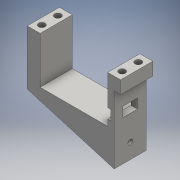
# Autodesk Inventor part: supportservopetitrobot
Saved by Autodesk Inventor 2016 (Build 200138000, 138)
## iProperties
Created: 2017-04-12
Part Number: supportservopetitrobot
Material: Générique
Document SubType Name: Modeling
Designer: Galileo
Density: 1 g/cm^3
Appearance: Par défaut
Author: Galileo
Autodesk Inventor part; units mm, degrees
ref_plane "YZ Plane" through (0, 0, 0) normal (1, 0, 0) x (0, 1, 0)
ref_plane "XZ Plane" through (0, 0, 0) normal (0, 1, 0) x (-1, 0, 0)
ref_plane "XY Plane" through (0, 0, 0) normal (0, 0, 1) x (1, 0, 0)
sketch "Esquisse1" plane through (0, 0, 0) normal (0, 1, 0) x (-1, 0, 0)
  line L0 (0, 0) -> (0, -8)
  line L1 (0, 0) -> (8, 0)
  line L2 (8, 0) -> (8, -29)
  line L3 (8, -29) -> (50, -29)
  line L4 (50, -29) -> (50, 0)
  line L5 (0, -8) -> (4, -8)
  line L6 (4, -8) -> (4, -50)
  line L7 (50, 0) -> (58, 0)
  line L8 (58, 0) -> (58, -34)
  line L9 (58, -34) -> (4, -50)
  dimension "d0" = 8
  dimension "d1" = 29
  dimension "d2" = 42
  dimension "d3" = 8
  dimension "d4" = 42
  dimension "d5" = 8
  dimension "d6" = 34
  dimension "d11" = 4
  dimension "d12" = 29
  constraints: 20 end point, 4 horizontal, 3 vertical, 2 perpendicular
  measures "d0" distance of L0.start L1.end
  measures "d1" distance of L1.end L2.end
  measures "d2" distance of L2.end L3.end
  measures "d3" distance of L0.start L0.end
  measures "d4" distance of L5.end L6.end
  measures "d5" distance of L4.end L7.end
  measures "d6" distance of L7.end L8.end
  measures "d11" distance of L0.end L5.end
  measures "d12" distance of L3.end L4.end
extrude "Extrusion1" add sketch "Esquisse1" along normal blind 20
sketch "Esquisse2" plane through (-58, 0, 0) normal (0, 0, 1) x (1, 0, 0)
  line L0 (0, 20) -> (8, 20) projected
  line L1 (0, 0) -> (8, 0) projected
  line L2 (0, 0) -> (0, 20) projected
  point P0 (58, 0)
  point P1 (4, 15)
  point P2 (4, 5)
  dimension "d15" = 10
  dimension "d17" = 5
  dimension "d18" = 4
  dimension "d19" = 4
  measures "d15" distance of point (4, 5) point (4, 15)
  measures "d17" distance from line of L1 point (4, 5)
  measures "d18" distance from line of L2 point (4, 15)
  measures "d19" distance from line of L2 point (4, 5)
hole "Perçage1" at (-54, 15, 0) at (-54, 5, 0) direction (0, 0, -1) diameter 4 depth 10 tip angle 118
sketch "Esquisse3" plane through (-8, 0, 0) normal (0, 0, 1) x (1, 0, 0)
  line L0 (0, 20) -> (8, 20) projected
  line L1 (8, 0) -> (8, 20) projected
  point P0 (4, 15)
  point P1 (4, 5)
  dimension "d27" = 10
  dimension "d28" = 5
  dimension "d29" = 4
  dimension "d30" = 4
  measures "d27" distance of point (4, 5) point (4, 15)
  measures "d28" distance from line of L0 point (4, 15)
  measures "d29" distance from line of L1 point (4, 5)
  measures "d30" distance from line of L1 point (4, 15)
hole "Perçage2" at (-4, 15, 0) at (-4, 5, 0) direction (0, 0, -1) diameter 4 depth 10 tip angle 118
sketch "Esquisse4" plane through (-4, 0, -8) normal (1, 0, 0) x (0, 0, -1)
  line L0 (42, 5) -> (27.5, 5)
  line L1 (27.5, 5) -> (27.5, 15)
  line L2 (27.5, 15) -> (42, 15)
  line L3 (42, 15) -> (42, 5)
  line L4 (0, 0) -> (42, 0) projected
  line L5 (42, 0) -> (42, 20) projected
  point P0 (-8, 0)
  dimension "d38" = 10
  dimension "d39" = 14.5
  dimension "d40" = 5
  dimension "d41" = 0
  constraints: 8 end point, 2 parallel, 1 horizontal, 1 perpendicular
  measures "d38" distance of L0.end L1.end
  measures "d39" distance between parallel lines of L3 L1
  measures "d40" distance between parallel lines of L0 L4
  measures "d41" distance between parallel lines of L5 L3
extrude "Extrusion2" cut sketch "Esquisse4" against normal blind 100
sketch "Esquisse5" plane through (-4, 15, -50) normal (0, -1, 0) x (1, 0, 0)
  line L0 (0, 42) -> (0, 0) projected
  line L1 (-4, 21) -> (0, 21)
  line L2 (0, 21) -> (0, 0)
  line L3 (0, 0) -> (-4, 0)
  line L4 (-4, 0) -> (-4, 21)
  point P0 (4, 50)
  constraints: 8 end point, 2 parallel, 1 horizontal, 1 perpendicular
extrude "Extrusion3" add sketch "Esquisse5" along normal blind 10
sketch "Esquisse6" plane through (-4, 0, -8) normal (1, 0, 0) x (0, 0, -1)
  line L0 (11, 5.5) -> (17, 5.5)
  line L1 (17, 5.5) -> (17, 14.5)
  line L2 (17, 14.5) -> (11, 14.5)
  line L3 (11, 14.5) -> (11, 5.5)
  line L4 (-8, 0) -> (-8, 20) projected
  line L5 (21, 20) -> (-8, 20) projected
  dimension "d49" = 19
  dimension "d50" = 25
  dimension "d51" = 9
  dimension "d52" = 5.5
  constraints: 8 end point, 2 parallel, 1 horizontal, 1 perpendicular
  measures "d49" distance between parallel lines of L4 L3
  measures "d50" distance between parallel lines of L4 L1
  measures "d51" distance between parallel lines of L2 L0
  measures "d52" distance between parallel lines of L5 L2
extrude "Extrusion4" cut sketch "Esquisse6" against normal blind 10
sketch "Esquisse7" plane through (-4, 0, -8) normal (1, 0, 0) x (0, 0, -1)
  line L0 (-8, 0) -> (-8, 20) projected
  line L1 (42, 15) -> (42, 5) projected
  line L2 (21, 0) -> (-8, 0) projected
  line L3 (42, 0) -> (26, 0) projected
  point P0 (1.5, 10)
  point P1 (32.5, 10)
  dimension "d55" = 9.5
  dimension "d56" = 9.5
  dimension "d57" = 10
  dimension "d58" = 10
  measures "d55" distance from line of L0 point (1.5, 10)
  measures "d56" distance from line of L1 point (32.5, 10)
  measures "d57" distance from line of L2 point (1.5, 10)
  measures "d58" distance from line of L3 point (32.5, 10)
hole "Perçage3" at (-4, 10, -9.5) at (-4, 10, -40.5) direction (-1, 0, 0) diameter 3 depth 20 tip angle 118
chamfer "Chanfrein2" distance 2 angle 45 1 edges at (-8, 10, -8)
sketch "Esquisse8" plane through (-8, 0, -29) normal (-1, 0, 0) x (0, 0, 1)
  line L0 (4, 14.5) -> (4, 5.5) projected
  line L1 (21, 0) -> (-21, 0) projected
  line L2 (4, 5.5) -> (10, 5.5)
  line L3 (10, 5.5) -> (10, 0)
  line L4 (10, 0) -> (4, 0)
  line L5 (4, 0) -> (4, 5.5)
  point P0 (29, 0)
  dimension "d69" = 6
  constraints: 8 end point, 2 parallel, 1 horizontal, 1 perpendicular, 1 point on line
  measures "d69" distance between parallel lines of L5 L3
extrude "Extrusion5" cut sketch "Esquisse8" against normal blind 2
chamfer "Chanfrein3" distance 4 angle 45 1 edges at (-8, 10, -50)
